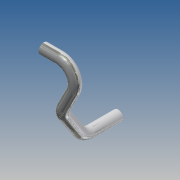
# Autodesk Inventor part: exhaust header right pipe 5
Saved by Autodesk Inventor 2013 (Build 170138000, 138)
## iProperties
Created: 2013-02-09
Part Number: exhaust header right pipe 5
Material: Steel
Document SubType Name: Modeling
Designer: zhaphod
Density: 1 g/cm^3
Author: zhaphod
Autodesk Inventor part; units mm, degrees
sketch "Sketch1" plane through (0, 0, 0) normal (1, 0, 0) x (0, 1, 0)
  line L0 (0, 0) -> (0, -185)
  line L1 (0, -185) -> (105.16, -332.225)
  line L2 (105.16, -332.225) -> (247.4, -332.225)
  line L3 (0, 0) -> (0, -165.1) construction
  line L4 (0, -165.1) -> (0, -71.825) construction
  line L5 (0, -71.825) -> (105.16, -52.775) construction
  line L6 (105.16, -52.775) -> (247.4, -52.775) construction
  dimension "d0" = 332.225
  dimension "d4" = 185
  dimension "d5" = 247.4
  dimension "d6" = 165.1
  dimension "d7" = 52.775
  dimension "d8" = 71.825
  dimension "d19" = 0
  dimension "d20" = 142.24
  constraints: 14 end point, 3 vertical alignment, 2 perpendicular, 1 horizontal
  measures "d0" distance from line of L2 L0.start
  measures "d4" distance of L0.end L0.start
  measures "d5" horizontal distance of L0.start L2.end
  measures "d6" distance of L0.start L3.end
  measures "d7" distance from line of L6 L0.start
  measures "d8" distance of L4.end L0.start
  measures "d19" horizontal distance of L0.end L0.start
  measures "d20" distance of L1.end L2.end
ref_plane "Work Plane1" through (165.1, 0, 0) normal (1, 0, 0) x (0, 1, 0)
ref_plane "Work Plane2" through (71.825, 0, 0) normal (1, 0, 0) x (0, 1, 0)
ref_plane "Work Plane3" through (52.775, 0, 0) normal (1, 0, 0) x (0, 1, 0)
sketch "Sketch2" plane through (165.1, 0, 0) normal (1, 0, 0) x (0, 1, 0)
  point P0 (0, 0)
  point P1 (0, 0)
sketch "Sketch3" plane through (71.825, 0, 0) normal (1, 0, 0) x (0, 1, 0)
  point P0 (0, 0)
  point P1 (0, -185)
  point P2 (105.16, -332.225)
sketch "Sketch4" plane through (52.775, 0, 0) normal (1, 0, 0) x (0, 1, 0)
  point P0 (0, 0)
  point P1 (247.4, -332.225)
  point P2 (105.16, -332.225)
sketch "Sketch5" plane through (0, 0, 0) normal (1, 0, 0) x (0, 1, 0)
  circle A0 centre (0, 0) radius 20.6375
  circle A1 centre (0, 0) radius 19.0375
  dimension "d15" = 1.6
  dimension "d17" = 41.275
  constraints: 2 centre point, 2 coincident
  measures "d15" radial gap between concentric circles of A0 A1
  measures "d17" diameter of A0
sketch3d "3D Sketch1"
  line L0 (0, 0, 0) -> (64.5477, 0, 0)
  arc A0 (64.5477, 0, 0) -> (119.831, 0, -89.7857) centre (64.5477, 0, -61.9125) ccw
  line L1 (119.831, 0, -89.7857) -> (81.8787, 0, -165.0596)
  arc A1 (81.8787, 0, -165.0596) -> (69.4866, 12.9085, -203.0721) centre (105.334, 56.0639, -176.8854) ccw
  line L2 (69.4866, 12.9085, -203.0721) -> (56.1274, 86.654, -306.3164)
  arc A2 (56.1274, 86.654, -306.3164) -> (52.775, 137.1751, -332.225) centre (60.7199, 137.1751, -270.8244) ccw
  line L3 (52.775, 137.1751, -332.225) -> (52.775, 247.4, -332.225)
  dimension "d13" = 61.9125
  dimension "d14" = 61.9125
  dimension "d12" = 61.9125
  constraints: 2 vertical
sweep "Sweep1" add profiles "Sketch5" path "3D Sketch1"
equation "\"d13\" = d12"
equation "\"d14\" = d12"
equation "\"d9\" = d6"
equation "\"d10\" = d8"
equation "\"d11\" = d7"
body "Solid1"
